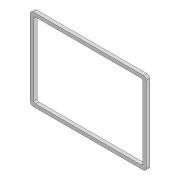
# Autodesk Inventor part: O-RING DASH 036 SQUARE
Saved by Autodesk Inventor 2020 (Build 240168000, 168)
## iProperties
Created: 2020-04-26
Part Number: O-RING DASH 036 SQUARE
Material: Generic
Document SubType Name: Modeling
Designer: John K
Density: 1 g/cm^3
Appearance: Default
Description: McM 4061T141
Author: John K
Autodesk Inventor part; units mm, degrees
ref_plane "YZ Plane" through (0, 0, 0) normal (1, 0, 0) x (0, 1, 0)
ref_plane "XZ Plane" through (0, 0, 0) normal (0, 1, 0) x (-1, 0, 0)
ref_plane "XY Plane" through (0, 0, 0) normal (0, 0, 1) x (1, 0, 0)
sketch "Sketch1" plane through (0, 0, 0) normal (0, 0, 1) x (1, 0, 0)
  line L0 (-28.575, -19.685) -> (28.575, -19.685)
  line L1 (28.575, -19.685) -> (28.575, 19.685)
  line L2 (28.575, 19.685) -> (-28.575, 19.685)
  line L3 (-28.575, 19.685) -> (-28.575, -19.685)
  line L4 (-28.575, -19.685) -> (28.575, 19.685) construction
  line L5 (28.575, -19.685) -> (-28.575, 19.685) construction
  line L6 (-30.353, 21.463) -> (30.353, 21.463)
  line L7 (30.353, 21.463) -> (30.353, -21.463)
  line L8 (30.353, -21.463) -> (-30.353, -21.463)
  line L9 (-30.353, -21.463) -> (-30.353, 21.463)
  point P0 (0, 0)
  dimension "d0" = 57.15
  dimension "d1" = 39.37
  dimension "d2" = 1.778
  constraints: 20 end point, 4 parallel, 2 midpoint, 2 perpendicular, 1 horizontal, 3 other
  measures "d0" distance of L2.end L1.end
  measures "d1" distance of L0.end L1.end
  measures "d2" distance between parallel lines of L2 L6
extrude "Extrusion1" add sketch "Sketch1" along normal mid plane 1.778
fillet "Fillet1" radius 1 4 edges at (-28.575, -19.685, 0) (-28.575, 19.685, 0) (28.575, 19.685, 0) (28.575, -19.685, 0)
fillet "Fillet1" radius 1.5 4 edges at (-30.353, 21.463, 0) (-30.353, -21.463, 0) (30.353, -21.463, 0) (30.353, 21.463, 0)
body "Solid1"
